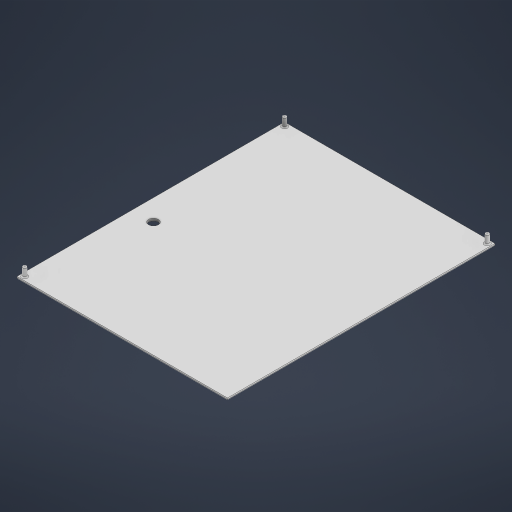
# Autodesk Inventor part: enclosure_lid
Saved by Autodesk Inventor 2023 (Build 270158000, 158)
## iProperties
Created: 2022-04-29
Part Number: enclosure_lid
Material: Generic
Document SubType Name: Modeling
Designer: Haroon Nawaz
Density: 1 g/cm^3
Appearance: Default
Author: Haroon Nawaz
Autodesk Inventor part; units mm, degrees
ref_plane "YZ Plane" through (0, 0, 0) normal (1, 0, 0) x (0, 1, 0)
ref_plane "XZ Plane" through (0, 0, 0) normal (0, 1, 0) x (-1, 0, 0)
ref_plane "XY Plane" through (0, 0, 0) normal (0, 0, 1) x (1, 0, 0)
sketch "Sketch1" plane through (0, 0, 0) normal (0, 1, 0) x (-1, 0, 0)
  line L0 (0, 0) -> (43.2562, 0)
  line L1 (43.2562, 0) -> (43.2562, -54.991)
  line L2 (43.2562, -54.991) -> (0, -54.991)
  line L3 (0, -54.991) -> (0, 0)
  dimension "d0" = 43.2562
  dimension "d1" = 54.991
  constraints: 8 end point, 2 parallel, 1 horizontal, 1 perpendicular
  measures "d0" distance of L1.end L2.end
  measures "d1" distance of L0.end L1.end
extrude "Extrusion1" add sketch "Sketch1" along normal blind 0.5
sketch "Sketch2" plane through (0, 0.5, 0) normal (0, 1, 0) x (1, 0, 0)
  circle A0 centre (-42.4688, 0.7874) radius 0.381
  circle A1 centre (-42.4688, 54.2036) radius 0.381
  circle A2 centre (-0.7874, 54.2036) radius 0.381
  circle A3 centre (-0.7874, 0.7874) radius 0.381
  point P0 (0, 0)
  dimension "d4" = 0.762
  dimension "d5" = 0.762
  dimension "d6" = 0.762
  dimension "d10" = 0.762
  constraints: 4 centre point, 4 coincident
  measures "d4" diameter of A0
  measures "d5" diameter of A1
  measures "d6" diameter of A2
  measures "d10" diameter of A3
extrude "Extrusion2" add sketch "Sketch2" along normal blind 1.905 contours A0 | A1 | A2
fillet "Fillet1" radius 0.2286 10 edges at (-42.8498, 2.405, -0.7874) (-42.8498, 2.405, -54.2036) (-1.1684, 2.405, -54.2036) (-1.1684, 0.5, -54.2036) (-42.8498, 0.5, -54.2036) (-42.8498, 0.5, -0.7874) (-21.6281, 0, 0) (0, 0, -27.4955) (-21.6281, 0, -54.991) (-43.2562, 0, -27.4955)
sketch "Sketch3" plane through (0, 0.5, 0) normal (0, 1, 0) x (1, 0, 0)
  line L0 (0, 54.991) -> (-43.2562, 54.991) projected
  line L1 (0, 54.991) -> (0, 25.019)
  line L2 (0, 54.991) -> (0, 0) projected
  line L3 (0, 25.019) -> (-2.8956, 25.019)
  line L4 (-43.2562, 25.019) -> (-40.3606, 25.019)
  line L5 (-40.3606, 25.019) -> (-39.3606, 25.019)
  point P0 (-38.9037, 23.6963)
  dimension "d11" = 29.972
  dimension "d12" = 2.8956
  dimension "d20" = 2.8956
  dimension "d21" = 1
  constraints: 8 end point, 3 point on line, 2 coincident, 1 horizontal, 1 perpendicular
  measures "d11" distance of L0.start L1.end
  measures "d12" distance of L1.end L3.end
  measures "d20" distance of L4.start L4.end
  measures "d21" distance of L4.end L5.end
hole "Hole1" at (-38.9037, 0.5, -23.6963) direction (0, -1, 0) diameter 2 end through all
body "Solid1"
